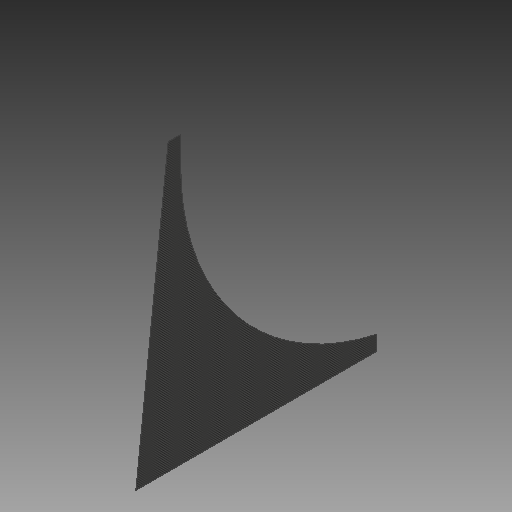
# Autodesk Inventor part: Side CFRP Cover
Saved by Autodesk Inventor 2019.4 (Build 234330000, 330)
## iProperties
Created: 2020-01-11
Part Number: Side CFRP Cover
Material: CFRP
Document SubType Name: Modeling
Designer: admin
Density: 1.43 g/cm^3
Appearance: Carbon Fiber
Mass: 21.6863 g
Surface Area: 1519.85 cm^2
Volume: 15.1653 cm^3
Author: admin
Autodesk Inventor part; units mm, degrees
ref_plane "YZ Plane" through (0, 0, 0) normal (1, 0, 0) x (0, 1, 0)
ref_plane "XZ Plane" through (0, 0, 0) normal (0, 1, 0) x (-1, 0, 0)
ref_plane "XY Plane" through (0, 0, 0) normal (0, 0, 1) x (1, 0, 0)
sketch "Sketch1" plane through (0, 0, 0) normal (1, 0, 0) x (0, 1, 0)
  circle A0 centre (-75.5115, -763.3089) radius 2.75 projected
  circle A1 centre (-75.5115, -743.3089) radius 2.75 projected
  circle A2 centre (-75.5115, -783.3089) radius 2.75 projected
  circle A3 centre (-50.5115, -332.8013) radius 2.75 projected
  circle A4 centre (-50.5115, -352.8013) radius 2.75 projected
  circle A5 centre (-50.5115, -312.8013) radius 2.75 projected
  circle A6 centre (396.4564, 25.2987) radius 9.5 projected
  circle A7 centre (354.4564, 24.2987) radius 9.5 projected
  circle A8 centre (19.2614, -184.11) radius 9.5 projected
  circle A9 centre (-77.2339, -682.9053) radius 9.5 projected
  circle A10 centre (232.0881, -190.7096) radius 9.5 projected
  circle A11 centre (119.788, -412.2936) radius 9.5 projected
  circle A12 centre (293.2722, -172.8055) radius 2.75 projected
  circle A13 centre (91.0811, -112.7413) radius 2.75 projected
  circle A14 centre (135.0252, -350.3913) radius 2.75 projected
  circle A15 centre (-58.8231, -530.2616) radius 2.75 projected
  circle A16 centre (103.4728, -547.5632) radius 2.75 projected
  circle A17 centre (-10.5755, -280.8639) radius 2.75 projected
  circle A18 centre (191.1752, -239.5993) radius 2.75 projected
  circle A19 centre (258.6786, -8.537) radius 2.75 projected
  circle A20 centre (87.1577, -682.8329) radius 9.5 projected
  circle A21 centre (150.2624, -288.489) radius 9.5 projected
  circle A22 centre (354.4564, -154.9013) radius 9.5 projected
  circle A23 centre (-40.4124, -377.6178) radius 9.5 projected
  circle A24 centre (162.9009, -41.3726) radius 9.5 projected
  circle A25 centre (396.4564, -155.9013) radius 9.5 projected
  arc A26 (27.4885, -793.3089) -> (107.4885, -713.3089) centre (27.4885, -713.3089) ccw projected
  line L0 (107.4885, -693.3089) -> (107.4885, -713.3089) projected
  arc A27 (108.9276, -669.36) -> (107.4885, -693.3089) centre (307.4885, -693.3089) ccw projected
  line L1 (108.9276, -669.36) -> (145.1113, -369.36) projected
  arc A28 (373.4564, -166.9013) -> (145.1113, -369.36) centre (373.4564, -396.9013) ccw projected
  line L2 (373.4564, -166.9013) -> (423.4564, -166.9013) projected
  line L3 (423.4564, -166.9013) -> (423.4564, 76.2987) projected
  line L4 (423.4564, 76.2987) -> (-93.5115, 134.6987) projected
  line L5 (-93.5115, 134.6987) -> (-93.5115, -299.8013) projected
  line L6 (-93.5115, -299.8013) -> (-66.5115, -299.8013) projected
  arc A29 (-63.5115, -302.8013) -> (-66.5115, -299.8013) centre (-66.5115, -302.8013) ccw projected
  line L7 (-63.5115, -302.8013) -> (-63.5115, -382.8013) projected
  arc A30 (-66.5115, -385.8013) -> (-63.5115, -382.8013) centre (-66.5115, -382.8013) ccw projected
  line L8 (-66.5115, -385.8013) -> (-93.5115, -385.8013) projected
  line L9 (-93.5115, -385.8013) -> (-93.5115, -732.3089) projected
  line L10 (-91.5115, -732.3089) -> (-93.5115, -732.3089) projected
  arc A31 (-88.5115, -735.3089) -> (-91.5115, -732.3089) centre (-91.5115, -735.3089) ccw projected
  line L11 (-88.5115, -793.3089) -> (-88.5115, -735.3089) projected
  line L12 (27.4885, -793.3089) -> (-88.5115, -793.3089) projected
  arc A32 (373.4564, 53.6541) -> (-66.5115, -299.8013) centre (373.4564, -396.9013) ccw
  line L13 (373.4564, 53.6541) -> (423.4564, 53.6541)
  circle A33 centre (414.4564, -53.7013) radius 2.75 projected
  circle A34 centre (414.4564, 16.2987) radius 2.75 projected
  circle A35 centre (414.4564, -123.7013) radius 2.75 projected
  circle A36 centre (-69.0393, -48.4336) radius 2.2 projected
  circle A37 centre (-19.0393, -48.4336) radius 2.2 projected
  circle A38 centre (-19.0393, -98.4336) radius 2.2 projected
  circle A39 centre (-69.0393, -98.4336) radius 2.2 projected
  constraints: 2 end point, 2 point on circle, 1 centre point, 1 coincident, 1 perpendicular, 1 point on line, 1 tangent
extrude "Extrusion1" add sketch "Sketch1" along normal blind 0.2 contours L13 A32 L6 L5 L4 L3 | A36 | A37 | A38 | A39
body "Solid1"
